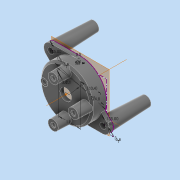
# Autodesk Inventor part: B1cover
Saved by Autodesk Inventor 2022 (Build 260153000, 153)
## iProperties
Created: 2024-04-23
Part Number: B1cover
Material: UHMW、黒
Document SubType Name: Modeling
Designer: ktamu
Density: 0.94 g/cm^3
Appearance: 滑らか - 黒
Author: ktamu
Autodesk Inventor part; units mm, degrees
ref_plane "YZ Plane" through (0, 0, 0) normal (1, 0, 0) x (0, 1, 0)
ref_plane "XZ Plane" through (0, 0, 0) normal (0, 1, 0) x (-1, 0, 0)
sketch "BASEscetch" plane through (0, 0, 0) normal (0, 0, 1) x (1, 0, 0)
  circle A0 centre (0, 0) radius 13.5
  circle A1 centre (0, 0) radius 12.4
  circle A2 centre (-11, 0) radius 1.05
  circle A3 centre (0, 0) radius 3
  circle A4 centre (0, 10.4) radius 1.05
  circle A5 centre (0, 10.4) radius 2.6
  circle A6 centre (0, 10.4) radius 2.45
  circle A7 centre (-11, 0) radius 1.8
  line L0 (11.970292, 5.423105) -> (12.970292, 5.423105) construction
  circle A8 centre (-13.290676, 10) radius 3.5
  circle A9 centre (-13.290676, 10) radius 2.8
  circle A10 centre (-13.290676, 10) radius 1.5
  circle A11 centre (13.530485, -10) radius 2.8
  circle A12 centre (13.530485, -10) radius 3.5
  circle A13 centre (13.530485, -10) radius 1.5
  line L1 (-13.479156, 10) -> (13.530485, 10)
  line L2 (13.530485, 10) -> (13.530485, -10)
  line L3 (13.530485, -10) -> (-13.479156, -10)
  line L4 (-13.479156, -10) -> (-13.479156, 10)
  line L5 (0, 13.5) -> (-13.290676, 13.5)
  line L6 (13.530485, -13.5) -> (0, -13.5)
  line L7 (13.530485, -10) -> (16.005359, -7.525126) construction
  line L8 (13.530485, -10) -> (17.030485, -10) construction
  line L9 (16.005359, -7.525126) -> (12.792684, -4.312451)
  line L10 (16.005359, -7.525126) -> (20.548768, -7.525126) construction
  line L11 (-13.290676, 10) -> (-15.76555, 7.525126)
  line L12 (-13.290676, 10) -> (-9.790676, 10) construction
  line L13 (-15.76555, 7.525126) -> (-12.731185, 4.490761)
  point P0 (-12.341818, -1.199802)
  point P1 (-12.341818, 1.199802)
  point P2 (-8.38296, 11.819025)
  point P3 (-8.381392, 11.506994)
  point P4 (10.65461, -8.36427)
  point P5 (16.930848, -13.995584)
  point P6 (-9.821799, 10.465716)
  point P7 (17.006973, -9.594987)
  point P8 (-9.796239, 10.197241)
  dimension "d0" = 27
  dimension "d1" = 24.8
  dimension "d2" = 2.1
  dimension "d3" = 11
  dimension "d4" = 6
  dimension "d11" = 2.1
  dimension "d12" = 5.2
  dimension "d13" = 4.9
  dimension "d14" = 0.5
  dimension "d29" = 3.6
  dimension "d40" = 7
  dimension "d41" = 5.6
  dimension "d42" = 3
  dimension "d43" = 7
  dimension "d44" = 5.6
  dimension "d45" = 3
  dimension "d46" = 45
  dimension "d47" = 135
  dimension "d48" = 135
  dimension "d75" = 10.4
  constraints: 28 end point, 14 centre point, 11 point on circle, 10 coincident, 6 horizontal, 3 equal length, 3 tangent, 2 parallel, 2 perpendicular
  measures "d0" diameter of A0
  measures "d1" diameter of A1
  measures "d2" diameter of A2
  measures "d3" distance of point (0, 0) A2.centre
  measures "d4" diameter of A3
  measures "d11" diameter of A4
  measures "d12" diameter of A5
  measures "d13" diameter of A6
  measures "d29" diameter of A7
  measures "d40" diameter of A8
  measures "d41" diameter of A9
  measures "d42" diameter of A10
  measures "d43" diameter of A12
  measures "d44" diameter of A11
  measures "d45" diameter of A13
  measures "d46" angle of L8 L7
  measures "d47" angle of L10 L9
  measures "d48" angle of L11 L12
  measures "d75" distance of point (0, 0) A4.centre
extrude "押し出し1" add sketch "BASEscetch" against normal blind 7.5 contours A0 A12 L3 A1 L1 | A0 A12 | L1 A1 A5 A0 | A0 L3 A1 | L1 A1 A7 L3 A0 L4 A8 | A1 A6 A5 | A8 A0 | A1 A6 | A1 A7 | A0 L4 picked at (-12.529021, 0)
extrude "押し出し3" add sketch "BASEscetch" against normal blind 2 contours L1 A5 A1 | A1 L3 A7 L1 A5 | A5 L1 A6 A1 | A5 L1 A6 | A1 L3 | A1 A5 L1 | A6 L1 A4 A1 | A1 A6 L1 A5 | A6 L1 A4 | A7 A1 | L1 A4 | A4 L1 picked at (-12.221693, -0.696084)
extrude "押し出し4" add sketch "BASEscetch" along normal blind 6.5 contours A5 L1 A6 A1 | A1 A6 A5 | A5 L1 A6 | A1 A6 L1 A5
extrude "押し出し5" add sketch "BASEscetch" along normal blind 6 contours A6 L1 A4 A1 | A1 A6 | A6 L1 A4
draft "面の勾配1" angle 1.9 pull direction (0, 0, 1) faces at (2.566331, 9.982931, 4.333333) fixed edges at (-2.6, 10.4, 6.5)
sketch "topScetch" plane through (0, 10.4, 6) normal (0, 0, 1) x (1, 0, 0)
  circle A0 centre (0, 0) radius 1.25
  circle A1 centre (0, 0) radius 2.45
  point P0 (0, -10.4)
  dimension "d20" = 2.5
  constraints: 2 centre point, 1 coincident
  measures "d20" diameter of A0
extrude "押し出し6" add sketch "topScetch" along normal blind 0.5
pattern_circular "円形状パターン1" count 3 over 180 about axis through (0, 0, 0) along (0, 0, -1) of "押し出し4", "押し出し6", "押し出し5", "面の勾配1"
chamfer "面取り1" distance 1 angle 45 1 edges at (-13.5, 0, 0)
extrude "押し出し7" add sketch "BASEscetch" along normal blind 0.04 contours A7 A1 | A1 A7
extrude "押し出し8" add sketch "BASEscetch" against normal blind 0.46 contours A1 A7 picked at (-12.529021, 0)
sketch "スケッチ3" plane through (0, 0, -7.5) normal (0, 0, -1) x (-1, 0, 0)
  point P0 (0, 0)
sketch "スケッチ4" plane through (0, 0, -7.5) normal (0, 0, -1) x (-1, 0, 0)
  point P0 (0, 0)
sketch "スケッチ5" plane through (0, 0, -7.5) normal (0, 0, -1) x (-1, 0, 0)
  point P0 (0, 0)
sketch "スケッチ6" plane through (0, 0, -7.5) normal (0, 0, -1) x (-1, 0, 0)
  point P0 (0, 0)
sketch "スケッチ7" plane through (0, 0, -7.5) normal (0, 0, -1) x (-1, 0, 0)
  point P0 (0, 0)
ref_plane "作業平面1" through (0, 0, -7.5) normal (0, 0, 1) x (1, 0, 0)
sketch "スケッチ8" plane through (0, 0, -7.5) normal (0, 0, 1) x (1, 0, 0)
  point P0 (0, 0)
sketch "seconbasescetch" plane through (0, 0, -7.5) normal (0, 0, 1) x (1, 0, 0)
  circle A0 centre (0, 0) radius 13.5
  circle A1 centre (0, 0) radius 12.4
  circle A2 centre (-11, 0) radius 1.05
  circle A3 centre (0, 0) radius 3
  circle A4 centre (0, 10.4) radius 1.05
  circle A5 centre (0, 10.4) radius 2.6
  circle A6 centre (0, 10.4) radius 2.45
  circle A7 centre (-11, 0) radius 1.8
  line L0 (11.970292, 5.423105) -> (12.970292, 5.423105) construction
  circle A8 centre (-13.290676, 10) radius 3.5
  circle A9 centre (-13.290676, 10) radius 2.8
  circle A10 centre (-13.290676, 10) radius 1.5
  circle A11 centre (13.530485, -10) radius 3.5
  circle A12 centre (13.530485, -10) radius 2.8
  circle A13 centre (13.530485, -10) radius 1.5
  line L1 (13.530485, -10) -> (-13.479156, -10)
  line L2 (-13.479156, -10) -> (-13.479156, 10)
  line L3 (-13.479156, 10) -> (13.530485, 10)
  line L4 (13.530485, 10) -> (13.530485, -10)
  line L5 (0, 13.5) -> (-13.290676, 13.5)
  line L6 (13.530485, -13.5) -> (0, -13.5)
  line L7 (13.530485, -10) -> (16.005359, -7.525126) construction
  line L8 (13.530485, -10) -> (17.030485, -10) construction
  line L9 (16.005359, -7.525126) -> (12.792684, -4.312451)
  line L10 (16.005359, -7.525126) -> (20.548768, -7.525126) construction
  line L11 (-13.290676, 10) -> (-15.76555, 7.525126)
  line L12 (-13.290676, 10) -> (-9.790676, 10) construction
  line L13 (-15.76555, 7.525126) -> (-12.731185, 4.490761)
  circle A14 centre (10.4, 0) radius 1.05
  circle A15 centre (10.4, 0) radius 1.05
  point P0 (-12.341818, -1.199802)
  point P1 (-12.341818, 1.199802)
  point P2 (-8.38296, 11.819025)
  point P3 (-8.381392, 11.506994)
  point P4 (10.65461, -8.36427)
  point P5 (16.930848, -13.995584)
  point P6 (-9.821799, 10.465716)
  point P7 (-9.796239, 10.197241)
  point P8 (17.006973, -9.594987)
  point P9 (10.246321, -8.789932)
  point P10 (11.409892, -7.215564)
  point P11 (-11.573427, 6.950237)
  point P12 (-9.884536, 9.194887)
  dimension "d50" = 27
  dimension "d51" = 24.8
  dimension "d52" = 2.1
  dimension "d53" = 11
  dimension "d54" = 6
  dimension "d55" = 2.1
  dimension "d56" = 5.2
  dimension "d57" = 4.9
  dimension "d58" = 0.5
  dimension "d59" = 3.6
  dimension "d60" = 7
  dimension "d61" = 5.6
  dimension "d62" = 3
  dimension "d63" = 7
  dimension "d64" = 5.6
  dimension "d65" = 3
  dimension "d66" = 45
  dimension "d67" = 135
  dimension "d68" = 135
  dimension "d76" = 10.4
  constraints: 28 end point, 15 centre point, 11 coincident, 11 point on circle, 6 horizontal, 3 equal length, 3 tangent, 2 parallel, 2 perpendicular, 1 concentric
  measures "d50" diameter of A0
  measures "d51" diameter of A1
  measures "d52" diameter of A2
  measures "d53" distance of point (0, 0) A2.centre
  measures "d54" diameter of A3
  measures "d55" diameter of A4
  measures "d56" diameter of A5
  measures "d57" diameter of A6
  measures "d59" diameter of A7
  measures "d60" diameter of A8
  measures "d61" diameter of A9
  measures "d62" diameter of A10
  measures "d63" diameter of A11
  measures "d64" diameter of A12
  measures "d65" diameter of A13
  measures "d66" angle of L8 L7
  measures "d67" angle of L10 L9
  measures "d68" angle of L11 L12
  measures "d76" distance of point (0, 0) A14.centre
extrude "押し出し9" add sketch "seconbasescetch" along normal blind 2 contours L9 L4 A11 A0 | L9 A11 L4 | A11 L1 A0 | A0 L3 A8 L5 | L1 A11 L6 A0 | A0 A8 L3 | A8 L2 L13 | A0 L13 L2 A8
extrude "押し出し10" add sketch "seconbasescetch" along normal blind 2 contours A11 L4 A12 L1 A0 | A11 L1 A12 L4 | L4 A13 L1 A12 | A12 L1 A13 L4 | A8 L3 A9 L11 | A0 A8 L2 A9 L3 | L11 A9 L2 A8 | L3 A10 L11 A9 | A9 L2 A10 L3 | L11 A10 L2 A9
sketch "seconbasescetch outline for 押し出し11" plane through (0, 0, -7.5) normal (0, 0, 1) x (1, 0, 0)
  circle A0 centre (-13.290676, 10) radius 3.5
  circle A1 centre (-13.290676, 10) radius 1.5
  arc A2 (10.246321, -8.789932) -> (11.409892, -7.215564) centre (13.530485, -10) ccw
  arc A3 (11.409892, -7.215564) -> (10.246321, -8.789932) centre (0, 0) cw
  circle A4 centre (13.530485, -10) radius 1.5
extrude "押し出し11" add sketch "seconbasescetch outline for 押し出し11" against normal blind 20.25 draft -2.45
